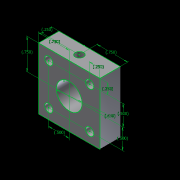
# Autodesk Inventor part: alignmentplate
Saved by Autodesk Inventor 2012 (Build 160160000, 160)
## iProperties
Created: 2011-10-12
Part Number: alignmentplate
Material: Default
Document SubType Name: Modeling
Designer: shane
Density: 1 g/cm^3
Author: shane
Autodesk Inventor part; units mm, degrees
ref_plane "YZ Plane" through (0, 0, 0) normal (1, 0, 0) x (0, 1, 0)
ref_plane "XZ Plane" through (0, 0, 0) normal (0, 1, 0) x (-1, 0, 0)
ref_plane "XY Plane" through (0, 0, 0) normal (0, 0, 1) x (1, 0, 0)
sketch "Sketch1" plane through (0, 0, 0) normal (0, 0, 1) x (1, 0, 0)
  line L0 (-15.8683, 12.6347) -> (22.2317, 12.6347)
  line L1 (22.2317, 12.6347) -> (22.2317, -25.4653)
  line L2 (22.2317, -25.4653) -> (-15.8683, -25.4653)
  line L3 (-15.8683, -25.4653) -> (-15.8683, 12.6347)
  point P0 (0, 0)
  dimension "d0" = 38.1
  dimension "d1" = 38.1
  constraints: 8 end point, 2 parallel, 1 horizontal, 1 perpendicular
  measures "d0" distance of L1.end L2.end
  measures "d1" distance of L0.end L1.end
extrude "Extrusion1" add sketch "Sketch1" along normal blind 12.7
hole "Hole1" at (3.1817, -6.4153, 12.7) direction (0, 0, -1) diameter 16 end through all
hole "Hole2" at (-9.5183, 6.2847, 12.7) direction (0, 0, -1) diameter 5.08 end through all
hole "Hole3" at (15.8817, 6.2847, 12.7) direction (0, 0, -1) diameter 5.08 end through all
hole "Hole4" at (-9.5183, -19.1153, 12.7) direction (0, 0, -1) diameter 5.08 end through all
hole "Hole5" at (15.8817, -19.1153, 12.7) direction (0, 0, -1) diameter 5.08 end through all
hole "Hole6" at (3.1817, 12.6347, 6.35) direction (0, -1, 0) diameter 5.08 depth 12.7 tip angle 118
sketch "Sketch2" plane through (0, 0, 12.7) normal (0, 0, 1) x (1, 0, 0)
  circle A0 centre (15.8817, -19.1153) radius 2.54 projected
  circle A1 centre (-9.5183, -19.1153) radius 2.54 projected
  circle A2 centre (15.8817, 6.2847) radius 2.54 projected
  circle A3 centre (-9.5183, 6.2847) radius 2.54 projected
  circle A4 centre (3.1817, -6.4153) radius 8 projected
  line L0 (22.2317, 12.6347) -> (22.2317, -25.4653) projected
  line L1 (-15.8683, 12.6347) -> (22.2317, 12.6347) projected
  line L2 (-15.8683, -25.4653) -> (-15.8683, 12.6347) projected
  line L3 (22.2317, -25.4653) -> (-15.8683, -25.4653) projected
  point P0 (0, 0)
  dimension "d58" = 6.35
  dimension "d59" = 6.35
  dimension "d60" = 19.05
  dimension "d61" = 19.05
  dimension "d64" = 16
  dimension "d65" = 12.7
  dimension "d66" = 12.7
  dimension "d67" = 12.7
  measures "d58" distance from line of L0 A2.centre
  measures "d59" distance from line of L1 A2.centre
  measures "d60" distance from line of L2 A4.centre
  measures "d61" distance from line of L1 A4.centre
  measures "d64" diameter of A4
  measures "d65" horizontal distance of A3.centre A4.centre
  measures "d66" horizontal distance of A1.centre A4.centre
  measures "d67" horizontal distance of A3.centre A4.centre
sketch "Sketch3" plane through (-15.8683, 12.6347, 0) normal (0, 1, 0) x (1, 0, 0)
  circle A0 centre (19.05, -6.35) radius 2.54 projected
  line L0 (0, -12.7) -> (38.1, -12.7) projected
  line L1 (38.1, 0) -> (38.1, -12.7) projected
  line L2 (0, 0) -> (38.1, 0) projected
  line L3 (0, 0) -> (0, -12.7) projected
  point P0 (15.8683, 0)
  dimension "d62" = 6.35
  dimension "d63" = 19.05
  measures "d62" distance from line of L2 A0.centre
  measures "d63" distance from line of L1 A0.centre
body "Solid1"
